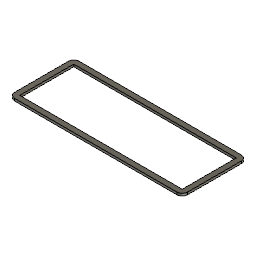
sourcefiles (Autodesk Fusion 360 design; units mm, degrees)
Autodesk Fusion 360 part; units mm, degrees
sketch "Sketch1" plane through (0, 0, 0) normal (0, 0, 1) x (1, 0, 0)
  line L0 (11, 0) -> (349.815, 0)
  line L1 (360.815, 11) -> (360.815, 123.629)
  line L2 (349.815, 134.629) -> (11, 134.629)
  line L3 (0, 123.629) -> (0, 11)
  arc A0 (11, 134.629) -> (0, 123.629) centre (11, 123.629) ccw
  arc A1 (0, 11) -> (11, 0) centre (11, 11) ccw
  arc A2 (349.815, 0) -> (360.815, 11) centre (349.815, 11) ccw
  arc A3 (360.815, 123.629) -> (349.815, 134.629) centre (349.815, 123.629) ccw
  line L4 (349.815, 11) -> (11, 11)
  line L5 (11, 11) -> (11, 123.629)
  line L6 (11, 123.629) -> (349.815, 123.629)
  line L7 (349.815, 123.629) -> (349.815, 11)
  dimension "d1" = 360.815
  dimension "d2" = 134.629
  dimension "d3" = 11
  dimension "d4" = 11
  dimension "d5" = 11
  dimension "d6" = 11
  constraint horizontal L0
  constraint vertical L1
  constraint horizontal L2
  constraint vertical L3
  constraint tangent L2 A0
  constraint tangent L3 A0
  constraint tangent L3 A1
  constraint tangent L0 A1
  constraint tangent L1 A2
  constraint tangent L0 A2
  constraint tangent L2 A3
  constraint tangent L1 A3
  constraint horizontal L4
  constraint vertical L5
  constraint horizontal L6
  constraint vertical L7
  constraint coincident A0.centre L5.end
  constraint coincident A2.centre L4.start
  measures "d1" distance of L1 L3
  measures "d2" distance of L0 L2
  measures "d3" radius of A0
  measures "d4" radius of A1
  measures "d5" radius of A2
  measures "d6" radius of A3
extrude "Extrude1" add sketch "Sketch1" along normal blind 5
